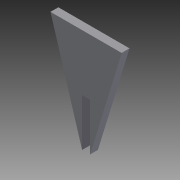
# Autodesk Inventor part: brace03
Saved by Autodesk Inventor 2013 (Build 170138000, 138)
## iProperties
Created: 2013-09-17
Part Number: brace03
Material: Generic
Document SubType Name: Modeling
Designer: Nano
Density: 1 g/cm^3
Author: Nano
Autodesk Inventor part; units mm, degrees
ref_plane "YZ Plane" through (0, 0, 0) normal (1, 0, 0) x (0, 1, 0)
ref_plane "XZ Plane" through (0, 0, 0) normal (0, 1, 0) x (-1, 0, 0)
ref_plane "XY Plane" through (0, 0, 0) normal (0, 0, 1) x (1, 0, 0)
sketch "Sketch1" plane through (0, 0, 0) normal (0, 0, 1) x (1, 0, 0)
  line L0 (-3.175, -49.7295) -> (-3.175, -11.6295)
  line L1 (-3.175, -11.6295) -> (3.175, -11.6295)
  line L2 (3.175, -11.6295) -> (3.175, -49.7295)
  line L3 (3.175, -49.7295) -> (28.575, 33.5996)
  line L4 (28.575, 33.5996) -> (-28.575, 33.5996)
  line L5 (-28.575, 33.5996) -> (-3.175, -49.7295)
  line L6 (0, -0.0188) -> (0, -58.4605) construction
  point P0 (0, 0)
  dimension "d3" = 6.35
  dimension "d4" = 38.1
  dimension "d5" = 38.1
  dimension "d6" = 90
  dimension "d7" = 90
  dimension "d12" = 45.2291
  dimension "d13" = 57.15
  dimension "d14" = 83.3291
  dimension "d15" = 17.5367
  dimension "d16" = 3.175
  dimension "d17" = 33.6184
  dimension "d18" = 92.0601
  constraints: 14 end point, 1 parallel, 1 perpendicular, 1 other
  measures "d3" distance of L0.end L1.end
  measures "d4" distance of L0.start L0.end
  measures "d5" distance of L1.end L2.end
  measures "d6" angle of L0 L1
  measures "d7" angle of L1 L2
  measures "d12" distance between parallel lines of L4 L1
  measures "d13" distance of L3.end L4.end
  measures "d14" vertical distance of L2.end L3.end
  measures "d15" distance from line of point (0, 0) L3
  measures "d16" distance from line of point (0, 0) L2
  measures "d17" distance from line of L6.start L4
  measures "d18" distance from line of L6.end L4
extrude "Extrusion1" add sketch "Sketch1" along normal blind 6.35
body "Solid1"
